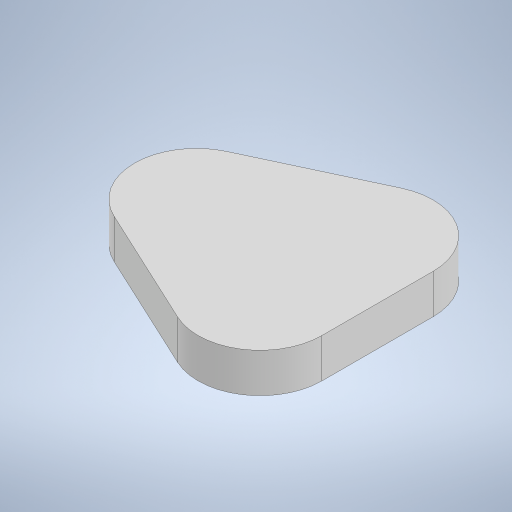
# Autodesk Inventor part: Magne_Cover
Saved by Autodesk Inventor 2024.3 (Build 283343000, 343)
## iProperties
Created: 2025-06-26
Part Number: Magne_Cover
Material: Generic
Document SubType Name: Modeling
Designer: 1
Density: 1 g/cm^3
Appearance: Default
Author: 1
Autodesk Inventor part; units mm, degrees
ref_plane "YZ Plane" through (0, 0, 0) normal (1, 0, 0) x (0, 1, 0)
ref_plane "XZ Plane" through (0, 0, 0) normal (0, 1, 0) x (-1, 0, 0)
ref_plane "XY Plane" through (0, 0, 0) normal (0, 0, 1) x (1, 0, 0)
sketch "Sketch1" plane through (0, 0, 0) normal (0, 1, 0) x (-1, 0, 0)
  line L0 (41.1155, 0) -> (-17.3761, 27.2751)
  line L1 (-17.3761, 27.2751) -> (-17.3761, -27.2751)
  line L2 (-17.3761, -27.2751) -> (41.1155, 0)
  circle A0 centre (-6.4761, -10.1655) radius 10.9
  circle A1 centre (-6.4761, 10.1655) radius 10.9
  circle A2 centre (15.3239, 0) radius 10.9
  circle A3 centre (0, 0) radius 17.3761
  line L3 (52.8138, 0) -> (-29.0745, 0) projected
  point P0 (-1.8696, 20.0443)
  point P1 (-17.3761, 10.1655)
  point P2 (-17.3761, -10.1655)
  point P3 (-1.8696, -20.0443)
  point P4 (19.9304, -9.8788)
  point P5 (19.9304, 9.8788)
  dimension "d0" = 50
  dimension "d1" = 21.8
  dimension "d2" = 32.7
  dimension "d3" = 21.8
  dimension "d4" = 21.8
  constraints: 9 tangent, 6 end point, 4 centre point, 1 coincident, 1 vertical, 1 other
  measures "d0" angle of L2 L0
  measures "d1" diameter of A0
  measures "d2" distance from line of L1 A2.centre
  measures "d3" diameter of A2
  measures "d4" diameter of A1
extrude "Extrusion1" add sketch "Sketch1" along normal blind 1 contours A2 A3 L0 | A2 L3 A3 | L2 A3 A2 | A2 A3 L3 | A3 A1 L0 | A3 A2 L3 A1 | A3 L3 A2 | L2 A0 A3 | A3 A0 L3 A2 | A2 L3 A3 | A1 A3 | A1 A0 A3 | A0 A3 | A3 A0 A1 | A1 A3 L1 | A1 L3 A3 | L3 A0 | A1 L3 | L1 A3 A0 | A3 L3 A0
sketch "Sketch2" plane through (0, 1, 0) normal (0, 1, 0) x (1, 0, 0)
  line L0 (17.3761, -10.1655) -> (17.3761, 10.1655) projected
  arc A0 (17.3761, 10.1655) -> (1.8696, 20.0443) centre (6.4761, 10.1655) ccw projected
  line L1 (1.8696, 20.0443) -> (-19.9304, 9.8788) projected
  arc A1 (-19.9304, 9.8788) -> (-19.9304, -9.8788) centre (-15.3239, 0) ccw projected
  line L2 (-19.9304, -9.8788) -> (1.8696, -20.0443) projected
  arc A2 (1.8696, -20.0443) -> (17.3761, -10.1655) centre (6.4761, -10.1655) ccw projected
  circle A3 centre (-15.3239, 0) radius 11.336
  circle A4 centre (6.4761, -10.1655) radius 11.336
  circle A5 centre (6.4761, 10.1655) radius 11.336
  line L3 (-20.1147, -10.2739) -> (1.6853, -20.4394)
  line L4 (-20.1147, 10.2739) -> (1.6853, 20.4394)
  line L5 (17.8121, -26) -> (17.8121, 10.1655)
  point P0 (0, 0)
  point P1 (17.8121, -10.1655)
  dimension "d9" = 22.672
  dimension "d7" = 22.672
  dimension "d8" = 22.672
  constraints: 6 end point, 4 point on circle, 4 tangent, 3 coincident, 2 centre point, 1 vertical, 4 other
  measures "d7" diameter of A3
  measures "d8" diameter of A5
extrude "Extrusion2" add sketch "Sketch2" against normal blind 1
sketch "Sketch3" plane through (0, 0, 0) normal (0, -1, 0) x (1, 0, 0)
  arc A0 (1.6853, -20.4394) -> (17.8121, -10.1655) centre (6.4761, -10.1655) ccw projected
  line L0 (17.8121, -10.1655) -> (17.8121, 10.1655) projected
  arc A1 (17.8121, 10.1655) -> (1.6853, 20.4394) centre (6.4761, 10.1655) ccw projected
  line L1 (1.6853, 20.4394) -> (-20.1147, 10.2739) projected
  arc A2 (-20.1147, 10.2739) -> (-20.1147, -10.2739) centre (-15.3239, 0) ccw projected
  line L2 (-20.1147, -10.2739) -> (1.6853, -20.4394) projected
  circle A3 centre (-15.3239, 0) radius 10.236
  circle A4 centre (6.4761, 10.1655) radius 10.236
  circle A5 centre (6.4761, -10.1655) radius 10.236
  line L3 (-19.6498, -9.277) -> (2.1502, -19.4425)
  line L4 (16.7121, -10.1655) -> (16.7121, 10.1655)
  line L5 (-19.6498, 9.277) -> (2.1502, 19.4425)
  point P0 (0, 0)
  point P1 (-8.7498, -14.3597)
  dimension "d17" = 1.1
  constraints: 6 end point, 6 point on circle, 6 tangent, 3 centre point, 3 coincident, 2 equal radius, 1 midpoint
  measures "d17" distance from line of L2 point (-8.75, -14.36)
extrude "Extrusion3" add sketch "Sketch3" along normal blind 5.1
sketch "Sketch4" plane through (0, -5.1, 0) normal (0, -1, 0) x (1, 0, 0)
  line L0 (1.6853, 20.4394) -> (-20.1147, 10.2739) projected
  arc A0 (17.8121, 10.1655) -> (1.6853, 20.4394) centre (6.4761, 10.1655) ccw projected
  line L1 (17.8121, -10.1655) -> (17.8121, 10.1655) projected
  arc A1 (1.6853, -20.4394) -> (17.8121, -10.1655) centre (6.4761, -10.1655) ccw projected
  line L2 (-20.1147, -10.2739) -> (1.6853, -20.4394) projected
  arc A2 (-20.1147, 10.2739) -> (-20.1147, -10.2739) centre (-15.3239, 0) ccw projected
  circle A3 centre (6.4761, -10.1655) radius 6.136
  circle A4 centre (6.4761, 10.1655) radius 6.136
  circle A5 centre (-15.3239, 0) radius 6.136
  line L3 (-17.917, -5.5611) -> (3.883, -15.7266)
  line L4 (12.6121, -10.1655) -> (12.6121, 10.1655)
  line L5 (3.883, 15.7266) -> (-17.917, 5.5611)
  point P0 (0, 0)
  dimension "d18" = 5.2
  constraints: 6 end point, 6 point on circle, 5 tangent, 3 centre point, 3 coincident, 2 equal radius, 1 vertical
  measures "d18" distance between parallel lines of L3 L2
extrude "Extrusion4" add sketch "Sketch4" along normal blind 1.1
body "Solid1"
